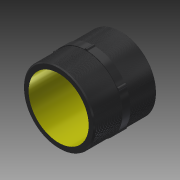
# Autodesk Inventor part: driftin cowboys
Saved by Autodesk Inventor 2013 SP2 (Build 170200200, 200)
## iProperties
Created: 2014-07-14
Part Number: driftin cowboys
Material: GFRP
Document SubType Name: Modeling
Designer: mrister
Density: 1.75 g/cm^3
Author: mrister
Autodesk Inventor part; units mm, degrees
ref_plane "YZ Plane" through (0, 0, 0) normal (1, 0, 0) x (0, 1, 0)
ref_plane "XZ Plane" through (0, 0, 0) normal (0, 1, 0) x (-1, 0, 0)
ref_plane "XY Plane" through (0, 0, 0) normal (0, 0, 1) x (1, 0, 0)
sketch "Sketch1" plane through (0, 0, 0) normal (0, 0, 1) x (1, 0, 0)
  circle A0 centre (0, 0) radius 36.5125
  circle A1 centre (0, 0) radius 43.6562
  dimension "d0" = 73.025
  dimension "d2" = 87.3125
  constraints: 2 centre point, 2 coincident
  measures "d0" diameter of A0
  measures "d2" diameter of A1
extrude "Extrusion1" add sketch "Sketch1" along normal mid plane 76.2
sketch "Sketch2" plane through (0, 0, 0) normal (0, 0, 1) x (1, 0, 0)
  circle A0 centre (0, 0) radius 44.45
  circle A1 centre (0, 0) radius 43.6562 projected
  circle A2 centre (0, 44.45) radius 1.5875
  line L0 (0, 44.45) -> (0, 0) construction
  circle A3 centre (-38.4948, 22.225) radius 1.5875
  circle A4 centre (-38.4948, -22.225) radius 1.5875
  circle A5 centre (0, -44.45) radius 1.5875
  circle A6 centre (38.4948, -22.225) radius 1.5875
  circle A7 centre (38.4948, 22.225) radius 1.5875
  dimension "d5" = 88.9
  dimension "d9" = 3.175
  dimension "d12" = 360
  constraints: 6 centre point, 2 end point, 1 coincident, 1 vertical, 1 vertical alignment, 15 other
  measures "d9" diameter of A2
extrude "Extrusion2" add sketch "Sketch2" along normal mid plane 9.525 contours A0 A6 A1 A7 | A7 A1 A0 | A0 A7 | A6 A0 | A0 A6 A1 | A7 A1 A2 A0 | A7 A1 | A0 A5 A1 A6 | A1 A6 | A2 A1 A0 | A0 A2 | A5 A0 | A0 A5 A1 | A2 A1 A3 A0 | A2 A1 | A0 A4 A1 A5 | A1 A5 | A3 A1 A0 | A0 A3 | A4 A0 | A0 A4 A1 | A3 A1 A4 A0 | A3 A1 | A1 A4
fillet "Fillet1" radius 1.5875 12 edges at (37.6767, 23.5854, 0) (39.2639, 20.8362, 0) (39.2639, -20.8362, 0) (37.6767, -23.5854, 0) (-1.5872, -44.4217, 0) (1.5872, -44.4217, 0) (1.5872, 44.4217, 0) (-1.5872, 44.4217, 0) (-37.6767, 23.5854, 0) (-39.2639, 20.8362, 0) (-39.2639, -20.8362, 0) (-37.6767, -23.5854, 0)
chamfer "Chamfer1" distance 1.5875 angle 45 2 edges at (-43.6562, 0, 38.1) (-43.6562, 0, -38.1)
sketch "Sketch3" plane through (0, 0, 0) normal (1, 0, 0) x (0, 1, 0)
  line L0 (43.6562, -36.5125) -> (43.6562, -4.7625) projected
  line L1 (43.6562, -50.4289) -> (43.6562, -51.2226)
  line L2 (43.6562, -51.2226) -> (42.8625, -50.8257)
  line L3 (42.8625, -50.8257) -> (43.6562, -50.4289)
  line L4 (42.8625, -50.8257) -> (43.6562, -50.8257) construction
  point P0 (0, 0)
  dimension "d18" = 0.7937
  constraints: 8 end point, 2 collinear, 1 horizontal, 1 midpoint, 1 perpendicular
  measures "d18" distance of L1.start L1.end
coil "Coil1" sketch "Sketch3" operation cut axis through (0, 0, -10) along (0, 0, 1) pitch 0.9525 turns 160 hand right
body "Solid1"
